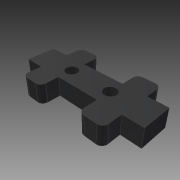
# Autodesk Inventor part: y_carriage_belt_mount_bed_holder
Saved by Autodesk Inventor 2014 (Build 180170000, 170)
## iProperties
Created: 2013-11-29
Part Number: y_carriage_belt_mount_bed_holder
Material: Plywood, Finish
Document SubType Name: Modeling
Designer: buben
Density: 0.552 g/cm^3
Appearance: Plywood - New
Author: buben
Subject: Laser Cutted
Autodesk Inventor part; units mm, degrees
ref_plane "YZ Plane" through (0, 0, 0) normal (1, 0, 0) x (0, 1, 0)
ref_plane "XZ Plane" through (0, 0, 0) normal (0, 1, 0) x (-1, 0, 0)
ref_plane "XY Plane" through (0, 0, 0) normal (0, 0, 1) x (1, 0, 0)
sketch "Sketch1" plane through (0, 0, 0) normal (0, 0, 1) x (1, 0, 0)
  line L0 (0, 0) -> (44, 0)
  line L1 (44, 0) -> (44, 10)
  line L2 (44, 10) -> (0, 10)
  line L3 (0, 10) -> (0, 0)
  circle A0 centre (29.5, 5) radius 2.25
  circle A1 centre (14.5, 5) radius 2.25
  line L4 (14.5, 5) -> (29.5, 5) construction
  point P0 (0, 5)
  point P1 (22, 5)
  point P2 (22, 10)
  dimension "d0" = 10
  dimension "d1" = 44
  dimension "d2" = 4.5
  dimension "d13" = 4.5
  dimension "d14" = 15
  constraints: 10 end point, 3 midpoint, 2 centre point, 2 parallel, 2 perpendicular, 1 horizontal, 1 horizontal alignment, 1 vertical alignment
  measures "d0" distance of L2.end L0.start
  measures "d1" distance of L0.start L0.end
  measures "d2" diameter of A0
  measures "d13" diameter of A1
  measures "d14" distance of L4.start L4.end
extrude "Extrusion3" add sketch "Sketch1" along normal blind 6.5
sketch "Sketch3" plane through (0, 0, 6.5) normal (0, 0, 1) x (1, 0, 0)
  line L0 (0, 0) -> (44, 0) projected
  line L1 (44, 10) -> (0, 10) projected
  line L2 (6.5, 10) -> (14.5, 10)
  line L3 (14.5, 10) -> (14.5, 14.5)
  line L4 (12.5, 16.5) -> (8.5, 16.5)
  line L5 (6.5, 14.5) -> (6.5, 10)
  line L6 (29.5, 10) -> (37.5, 10)
  line L7 (37.5, 10) -> (37.5, 14.5)
  line L8 (35.5, 16.5) -> (31.5, 16.5)
  line L9 (29.5, 14.5) -> (29.5, 10)
  line L10 (6.5, 0) -> (14.5, 0)
  line L11 (14.5, 0) -> (14.5, -4.5)
  line L12 (12.5, -6.5) -> (8.5, -6.5)
  line L13 (6.5, -4.5) -> (6.5, 0)
  line L14 (29.5, 0) -> (37.5, 0)
  line L15 (37.5, 0) -> (37.5, -4.5)
  line L16 (35.5, -6.5) -> (31.5, -6.5)
  line L17 (29.5, -4.5) -> (29.5, 0)
  arc A0 (8.5, 16.5) -> (6.5, 14.5) centre (8.5, 14.5) ccw
  arc A1 (14.5, 14.5) -> (12.5, 16.5) centre (12.5, 14.5) ccw
  arc A2 (31.5, 16.5) -> (29.5, 14.5) centre (31.5, 14.5) ccw
  arc A3 (37.5, 14.5) -> (35.5, 16.5) centre (35.5, 14.5) ccw
  arc A4 (6.5, -4.5) -> (8.5, -6.5) centre (8.5, -4.5) ccw
  arc A5 (12.5, -6.5) -> (14.5, -4.5) centre (12.5, -4.5) ccw
  arc A6 (29.5, -4.5) -> (31.5, -6.5) centre (31.5, -4.5) ccw
  arc A7 (35.5, -6.5) -> (37.5, -4.5) centre (35.5, -4.5) ccw
  line L18 (14.5, 12.5251) -> (29.5, 12.5251) construction
  point P0 (22, 12.5251)
  point P1 (22, 10)
  dimension "d17" = 2
  dimension "d18" = 8
  dimension "d19" = 8
  dimension "d20" = 6.5
  dimension "d21" = 6.5
  dimension "d22" = 15
  constraints: 34 end point, 16 point on circle, 16 tangent, 8 centre point, 8 parallel, 7 equal radius, 6 collinear, 6 point on line, 5 perpendicular, 4 horizontal, 2 midpoint, 1 vertical alignment
  measures "d17" radius of A0
  measures "d18" distance between parallel lines of L3 L5
  measures "d19" distance between parallel lines of L7 L9
  measures "d20" distance between parallel lines of L0 L12
  measures "d21" distance between parallel lines of L1 L4
  measures "d22" distance between parallel lines of L9 L3
extrude "Extrusion4" add sketch "Sketch3" against normal blind 6.5
equation "\"d20\" = d21"
body "Solid2"
